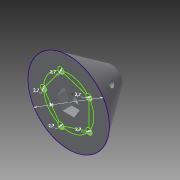
# Autodesk Inventor part: motorSupportShaft
Saved by Autodesk Inventor 2014 SP2 (Build 180246200, 246)
## iProperties
Created: 2020-04-08
Part Number: motorSupportShaft
Material: Generic
Document SubType Name: Sheet Metal
Designer: GauchoHP
Density: 1 g/cm^3
Sheet Metal Rule: Default_mm
Appearance: Default
Author: GauchoHP
Autodesk Inventor part; units mm, degrees
ref_plane "YZ Plane" through (0, 0, 0) normal (1, 0, 0) x (0, 1, 0)
ref_plane "XZ Plane" through (0, 0, 0) normal (0, 1, 0) x (-1, 0, 0)
ref_plane "XY Plane" through (0, 0, 0) normal (0, 0, 1) x (1, 0, 0)
sketch "Sketch1" plane through (0, 0, 0) normal (0, 1, 0) x (-1, 0, 0)
  circle A0 centre (0, 0) radius 18
  line L0 (10.3065, -1.0922) -> (4.2236, -9.4646)
  line L1 (2.1462, -10.1396) -> (-7.6962, -6.9416)
  line L2 (-8.9801, -5.1744) -> (-8.9801, 5.1744)
  line L3 (-7.6962, 6.9416) -> (2.1462, 10.1396)
  line L4 (4.2236, 9.4646) -> (10.3065, 1.0922)
  circle A1 centre (3.4301, 10.5567) radius 1.35
  circle A2 centre (11.1, 0) radius 1.35
  circle A3 centre (-8.9801, 6.5244) radius 1.35
  circle A4 centre (-8.9801, -6.5244) radius 1.35
  circle A5 centre (3.4301, -10.5567) radius 1.35
  arc A6 (11.0179, 1.3475) -> (4.6863, 10.0622) centre (0, 0) ccw
  arc A7 (4.6863, -10.0622) -> (11.0179, -1.3475) centre (0, 0) ccw
  arc A8 (-8.1216, -7.5663) -> (2.1232, -10.8951) centre (0, 0) ccw
  arc A9 (2.1232, 10.8951) -> (-8.1216, 7.5663) centre (0, 0) ccw
  arc A10 (-9.7057, 5.386) -> (-9.7057, -5.386) centre (0, 0) ccw
  dimension "d0" = 36
  dimension "d2" = 2.7
  dimension "d3" = 2.7
  dimension "d4" = 2.7
  dimension "d5" = 2.7
  dimension "d6" = 2.7
  constraints: 30 point on circle, 11 centre point, 10 end point, 3 coincident, 6 other
  measures "d0" diameter of A0
  measures "d2" diameter of A1
  measures "d3" diameter of A2
  measures "d4" diameter of A3
  measures "d5" diameter of A4
  measures "d6" diameter of A5
extrude "Extrusion1" add sketch "Sketch1" along normal blind 19 contours A0 | A2 A7 A5 L0 | L0 A5 L1 A4 L2 A3 L3 A1 L4 A2 | A2 | A5 | L4 A1 A6 A2 | A5 A8 A4 L1 | A1 | A4 | L3 A3 A9 A1 | A3 | A10 A3 L2 A4
sketch "Sketch3" plane through (0, 0, 0) normal (0, -1, 0) x (1, 0, 0)
  circle A0 centre (0, 0) radius 18 projected
  line L0 (-5.1962, 0) -> (-2.5981, 4.5)
  line L1 (-2.5981, 4.5) -> (2.5981, 4.5)
  line L2 (2.5981, 4.5) -> (5.1962, 0)
  line L3 (5.1962, 0) -> (2.5981, -4.5)
  line L4 (2.5981, -4.5) -> (-2.5981, -4.5)
  line L5 (-2.5981, -4.5) -> (-5.1962, 0)
  dimension "d23" = 9
  constraints: 12 end point, 1 coincident, 13 other
  measures "d23" distance between parallel lines of L3 L0
extrude "Extrusion3" cut sketch "Sketch3" against normal blind 4 contours L0 L1 L2 L3 L4 L5
sketch "Sketch4" plane through (0, 4, 0) normal (0, -1, 0) x (1, 0, 0)
  circle A0 centre (0, 0) radius 2.75
  dimension "d26" = 5.5
  constraints: 1 centre point, 1 coincident
  measures "d26" diameter of A0
extrude "Extrusion4" cut sketch "Sketch4" against normal blind 17
chamfer "Chamfer2" distance 13 distance2 19 1 edges at (18, 19, 0) measured on face at (-12.7157, 19, -1.6553)
extrude "Extrusion5" cut sketch "Sketch1" along normal blind 14 contours A2 | A5 | A1 | A4 | A3
equation "\"BendRadius\" = Thickness"
equation "\"BendReliefWidth\" = Thickness"
equation "\"BendReliefDepth\" = 0.5 * Thickness"
equation "\"CornerReliefSize\" = 4 * Thickness"
equation "\"MinimumRemnant\" = 2 * Thickness"
equation "\"TransitionRadius\" = BendRadius"
equation "\"JacobiRadiusSize\" = BendRadius"
equation "\"GapSize\" = Thickness"
equation "\"Thickness\" = 0.5"
body "Solid1"
